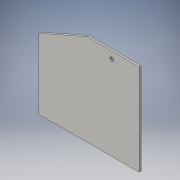
# Autodesk Inventor part: Bucket - door 2
Saved by Autodesk Inventor 2016 (Build 200138000, 138)
## iProperties
Created: 2016-01-14
Part Number: Bucket - door 2
Material: Generic
Document SubType Name: Modeling
Designer: TimB
Density: 1 g/cm^3
Appearance: Default
Author: TimB
Autodesk Inventor part; units mm, degrees
ref_plane "YZ Plane" through (0, 0, 0) normal (1, 0, 0) x (0, 1, 0)
ref_plane "XZ Plane" through (0, 0, 0) normal (0, 1, 0) x (-1, 0, 0)
ref_plane "XY Plane" through (0, 0, 0) normal (0, 0, 1) x (1, 0, 0)
sketch "Sketch1" plane through (0, 0, 0) normal (0, 0, 1) x (1, 0, 0)
  line L0 (72.5, 63.5) -> (-72.5, 63.5)
  line L1 (72.5, 63.5) -> (-72.5, -63.5) construction
  line L2 (-72.5, 63.5) -> (72.5, -63.5) construction
  circle A0 centre (33.08, -58.41) radius 2.85 projected
  line L3 (72.5, 63.5) -> (72.5, -68.5)
  line L4 (-72.5, -38.1) -> (-3.32, -68.5)
  line L5 (-72.5, 63.5) -> (-72.5, -38.1)
  line L6 (-3.32, -68.5) -> (72.5, -68.5)
  point P0 (0, 0)
  dimension "d5" = 132
  dimension "d6" = 145
  constraints: 14 end point, 2 midpoint, 1 horizontal, 1 perpendicular, 1 vertical
  measures "d5" distance of L0.start L3.end
  measures "d6" distance of L0.start L0.end
extrude "Extrusion2" add sketch "Sketch1" along normal blind 3
body "Solid2"
